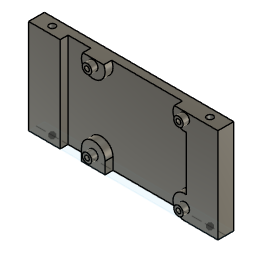
Wall_Raspberry (Autodesk Fusion 360 design; units mm, degrees)
Autodesk Fusion 360 part; units mm, degrees
sketch "Sketch1" plane through (0, 0, 0) normal (0, 0, 1) x (1, 0, 0)
  line L0 (0, 0) -> (120, 0)
  line L1 (120, 0) -> (120, 10)
  line L2 (120, 10) -> (0, 10)
  line L3 (0, 10) -> (0, 0)
  dimension "d1" = 120
  dimension "d2" = 10
  constraint horizontal L0
  constraint vertical L1
  constraint horizontal L2
  constraint vertical L3
  constraint coincident L0.start L3.end
  measures "d1" distance of L0.start L0.end
  measures "d2" distance of L0.start L2.end
extrude "Extrude1" add sketch "Sketch1" along normal blind 60
sketch "Sketch2" plane through (0, 0, 0) normal (0, 0, -1) x (1, 0, 0)
  line L0 (0, 0) -> (0, -10)
  line L1 (0, -10) -> (120, -10)
  line L2 (120, -10) -> (120, 0)
  line L3 (120, 0) -> (0, 0)
  line L4 (0, -5) -> (120, -5) construction
  point P0 (10, -5)
  point P1 (110, -5)
  dimension "d5" = 100
  dimension "d6" = 10
  constraint midpoint L0 L4.start
  constraint midpoint L2 L4.end
  constraint coincident L4 P0
  constraint coincident L4 P1
  measures "d5" distance of P0 P1
  measures "d6" distance of L2 P1
sketch "Sketch3" plane through (0, 0, 60) normal (0, 0, 1) x (-1, 0, 0)
  line L0 (0, -10) -> (0, 0)
  line L1 (0, 0) -> (-120, 0)
  line L2 (-120, 0) -> (-120, -10)
  line L3 (-120, -10) -> (0, -10)
  line L4 (0, -5) -> (-120, -5) construction
  point P0 (-10, -5)
  point P1 (-110, -5)
  dimension "d10" = 100
  dimension "d11" = 10
  constraint midpoint L0 L4.start
  constraint midpoint L2 L4.end
  constraint coincident L4 P0
  constraint coincident L4 P1
  measures "d10" distance of P0 P1
  measures "d11" distance of L2 P1
hole "Hole2" at (10, 5, 0) at (110, 5, 0) direction (0, 0, 1) diameter 4 depth 6 tip angle 180
hole "Hole3" at (10, 5, 60) at (110, 5, 60) direction (0, 0, -1) diameter 4 depth 6 tip angle 180
sketch "Sketch8" plane through (0, 10, 0) normal (0, 1, 0) x (-1, 0, 0)
  line L0 (-120, 0) -> (0, 0)
  line L1 (0, 0) -> (0, 60)
  line L2 (0, 60) -> (-120, 60)
  line L3 (-120, 60) -> (-120, 0)
  circle A0 centre (-99, 56.5) radius 1.35
  circle A1 centre (-41, 56.5) radius 1.35
  circle A2 centre (-99, 7.5) radius 1.35
  circle A3 centre (-41, 7.5) radius 1.35
  point P0 (-99, 56.5)
  point P1 (-41, 56.5)
  point P2 (-41, 7.5)
  point P3 (-99, 7.5)
  constraint coincident P0 A0.centre
  constraint coincident P1 A1.centre
  constraint coincident P2 A3.centre
  constraint coincident P3 A2.centre
hole "Hole5" at (99, 10, 56.5) at (41, 10, 56.5) at (99, 10, 7.5) at (41, 10, 7.5) direction (0, -1, 0) diameter 3 end through all counterbore diameter 5 counterbore depth 8
sketch "Sketch9" plane through (0, 0, 0) normal (0, -1, 0) x (1, 0, 0)
  circle A0 centre (99, 7.5) radius 1.5
  circle A1 centre (99, 56.5) radius 1.5
  circle A2 centre (41, 56.5) radius 1.5
  circle A3 centre (41, 7.5) radius 1.5
  line L0 (0, 0) -> (120, 0)
  line L1 (120, 0) -> (120, 60)
  line L2 (120, 60) -> (0, 60)
  line L3 (0, 60) -> (0, 0)
  circle A4 centre (41, 7.5) radius 3
  circle A5 centre (99, 7.5) radius 3
  circle A6 centre (99, 56.5) radius 3
  circle A7 centre (41, 56.5) radius 3
  dimension "d33" = 6
  dimension "d34" = 6
  dimension "d35" = 6
  dimension "d36" = 6
  constraint concentric A3 A4
  constraint concentric A0 A5
  constraint concentric A1 A6
  constraint concentric A2 A7
  measures "d33" diameter of A4
  measures "d34" diameter of A5
  measures "d35" diameter of A6
  measures "d36" diameter of A7
extrude "Extrude4" add sketch "Sketch9" along normal blind 4 contours A4 | A5 | A6 | A7
sketch "Sketch10" plane through (0, 0, 0) normal (0, -1, 0) x (1, 0, 0)
  circle A0 centre (41, 56.5) radius 3
  circle A1 centre (99, 7.5) radius 3
  circle A2 centre (41, 7.5) radius 3
  circle A3 centre (99, 56.5) radius 3
  line L0 (0, 0) -> (120, 0)
  line L1 (120, 0) -> (120, 60)
  line L2 (120, 60) -> (0, 60)
  line L3 (0, 60) -> (0, 0)
  line L4 (20, 0) -> (20, 60)
  arc A4 (100, 14.933) -> (100, 0.067) centre (99, 7.5) ccw
  arc A5 (34.3668, 60) -> (47.6332, 60) centre (41, 56.5) ccw
  line L5 (20, 60) -> (34.3668, 60)
  line L6 (47.6332, 60) -> (92.3668, 60)
  line L7 (33.5, 7.5) -> (33.5, 0)
  line L8 (48.5, 7.5) -> (48.5, 0)
  arc A6 (48.5, 7.5) -> (33.5, 7.5) centre (41, 7.5) ccw
  line L9 (100, 0) -> (48.5, 0)
  line L10 (33.5, 0) -> (20, 0)
  line L11 (100, 60) -> (100, 14.933)
  line L12 (100, 10.3284) -> (100, 4.6716)
  line L13 (100, 0.067) -> (100, 0)
  arc A7 (92.3668, 60) -> (100, 49.067) centre (99, 56.5) ccw
  dimension "d39" = 15
  dimension "d40" = 15
  dimension "d41" = 15
  dimension "d42" = 15
  dimension "d43" = 20
  dimension "d44" = 20
  constraint concentric A2 A6
  constraint concentric A3 A7
  constraint concentric A1 A4
  constraint concentric A0 A5
  constraint horizontal L5
  constraint vertical L11
  constraint horizontal L9
  constraint vertical L4
  constraint coincident L0 L9.start
  constraint coincident L2 L4.end
  constraint coincident A4.end L11
  constraint coincident L2 A5.end
  constraint coincident L2 A5.start
  constraint collinear L5 L6
  constraint coincident L7.end L9
  constraint perpendicular L7 L9
  constraint perpendicular L8 L9
  constraint collinear L9 L10
  constraint coincident A1 L12.start
  constraint collinear L11 L12
  constraint coincident A1 L12.end
  constraint collinear L12 L13
  constraint coincident L11 A7.end
  measures "d39" diameter of A6
  measures "d40" diameter of A7
  measures "d41" diameter of A4
  measures "d42" diameter of A5
  measures "d43" distance of L1 L11
  measures "d44" distance of L3 L4
extrude "Extrude5" cut sketch "Sketch10" against normal blind 5 contours L0 L2 L4 A4 A5 L5 L6 L7 L8 A6 L9 L10 L11 A7
equation "d6 = ( 120 mm - d5 ) / 2"
equation "d11 = ( 120 mm - d10 ) / 2"
equation "d34 = d33"
equation "d35 = d33"
equation "d36 = d33"
equation "d40 = d39"
equation "d41 = d39"
equation "d42 = d39"
